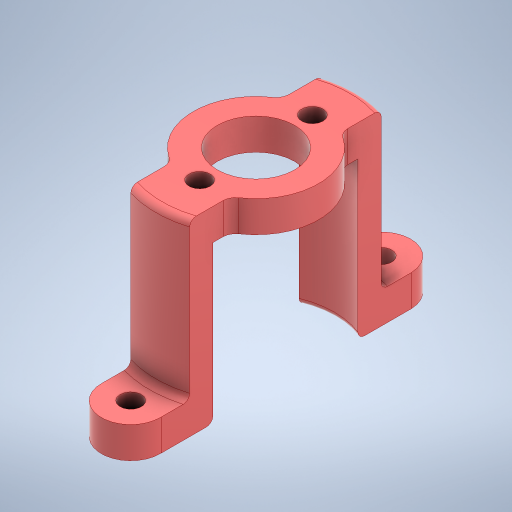
# Autodesk Inventor part: Th_3D_hn_1
Saved by Autodesk Inventor 2023 (Build 270158000, 158)
## iProperties
Created: 2020-11-15
Part Number: Th_3D_hn_1
Material: ABS プラスチック
Document SubType Name: Modeling
Designer: Haruka
Density: 1.06 g/cm^3
Appearance: 滑らか - 赤
Author: Haruka
Autodesk Inventor part; units mm, degrees
ref_plane "YZ Plane" through (0, 0, 0) normal (1, 0, 0) x (0, 1, 0)
ref_plane "XZ Plane" through (0, 0, 0) normal (0, 1, 0) x (-1, 0, 0)
ref_plane "XY Plane" through (0, 0, 0) normal (0, 0, 1) x (1, 0, 0)
sketch "スケッチ1" plane through (0, 0, 0) normal (0, 1, 0) x (-1, 0, 0)
  line L0 (0, 0) -> (0, -20) construction
  line L1 (0, 0) -> (0, 20) construction
  circle A0 centre (0, 20) radius 1.7
  circle A1 centre (0, -20) radius 1.7
  circle A2 centre (0, 20) radius 4.7
  circle A3 centre (0, -20) radius 4.7
  line L2 (4.698231, 19.871077) -> (4.7, -19.999792)
  line L3 (-4.697377, 19.843003) -> (-4.697377, -20.156997)
  circle A4 centre (0, 0) radius 12.5
  point P0 (-4.697377, 11.58381)
  point P1 (4.698599, 11.583314)
  point P2 (4.699627, -11.582897)
  point P3 (-4.697377, -11.58381)
  dimension "d0" = 20
  dimension "d1" = 20
  dimension "d2" = 3.4
  dimension "d3" = 3.4
  dimension "d5" = 3
  dimension "d6" = 3
  dimension "d7" = 25
  constraints: 8 end point, 5 centre point, 4 point on circle, 3 coincident, 3 vertical, 1 tangent
  measures "d0" distance of L0.start L0.end
  measures "d1" distance of L0.start L1.end
  measures "d2" diameter of A0
  measures "d3" diameter of A1
  measures "d5" radial gap between concentric circles of A0 A2
  measures "d6" radial gap between concentric circles of A3 A1
  measures "d7" diameter of A4
sketch "スケッチ1 outline for 押し出し1" plane through (0, 0, 0) normal (0, 1, 0) x (-1, 0, 0)
  arc A0 (-4.697377, 11.58381) -> (4.698599, 11.583314) centre (0, 0) cw
  line L0 (-4.697377, 19.843003) -> (-4.697377, 11.58381)
  line L1 (4.698599, 11.583314) -> (4.698231, 19.871077)
  arc A1 (4.698231, 19.871077) -> (-4.697377, 19.843003) centre (0, 20) ccw
  circle A2 centre (0, 20) radius 1.7
  arc A3 (-4.697377, -20.156997) -> (4.7, -19.999792) centre (0, -20) ccw
  line L2 (-4.697377, -11.58381) -> (-4.697377, -20.156997)
  line L3 (4.7, -19.999792) -> (4.699627, -11.582897)
  arc A4 (4.699627, -11.582897) -> (-4.697377, -11.58381) centre (0, 0) cw
  circle A5 centre (0, -20) radius 1.7
extrude "押し出し1" add sketch "スケッチ1 outline for 押し出し1" along normal blind 5
sketch "スケッチ2" plane through (0, 5, 0) normal (0, 1, 0) x (1, 0, 0)
  line L0 (-4.698599, -11.583314) -> (-4.698231, -19.871077)
  arc A0 (-4.698231, -19.871077) -> (4.697377, -19.843003) centre (0, -20) ccw
  line L1 (4.697377, -19.843003) -> (4.697377, -11.58381)
  arc A1 (-4.698599, -11.583314) -> (4.697377, -11.58381) centre (0, 0) ccw
  circle A2 centre (0, -20) radius 1.7
  arc A3 (4.697377, 20.156997) -> (-4.7, 19.999792) centre (0, 20) ccw
  line L2 (-4.7, 19.999792) -> (-4.699627, 11.582897)
  arc A4 (4.697377, 11.58381) -> (-4.699627, 11.582897) centre (0, 0) ccw
  line L3 (4.697377, 11.58381) -> (4.697377, 20.156997)
  circle A5 centre (0, 20) radius 1.7
  circle A6 centre (0, 0) radius 16
  point P0 (4.697377, 15.294922)
  point P1 (-4.699791, 15.294181)
  point P2 (-4.698434, -15.294598)
  point P3 (4.697377, -15.294922)
  dimension "d10" = 32
  constraints: 1 centre point, 1 coincident
  measures "d10" diameter of A6
extrude "押し出し2" add sketch "スケッチ2" along normal blind 20 contours A1 L1 A6 L0 | A6 L3 A4 L2
sketch "スケッチ3" plane through (0, 25, 0) normal (0, 1, 0) x (1, 0, 0)
  line L0 (-4.698599, -11.583314) -> (-4.698434, -15.294598)
  arc A0 (-4.698434, -15.294598) -> (4.697377, -15.294922) centre (0, 0) ccw
  line L1 (4.697377, -15.294922) -> (4.697377, -11.58381)
  arc A1 (-4.698599, -11.583314) -> (4.697377, -11.58381) centre (0, 0) ccw
  line L2 (-4.699791, 15.294181) -> (-4.699627, 11.582897)
  arc A2 (4.697377, 11.58381) -> (-4.699627, 11.582897) centre (0, 0) ccw
  line L3 (4.697377, 11.58381) -> (4.697377, 15.294922)
  arc A3 (4.697377, 15.294922) -> (-4.699791, 15.294181) centre (0, 0) ccw
  line L4 (-4.6, -11.583314) -> (-4.6, 11.582897)
  line L5 (4.697377, -11.58381) -> (4.697377, 11.58381)
  circle A4 centre (0, 0) radius 10
  point P0 (-4.699504, 8.826928)
  point P1 (-4.698721, -8.827345)
  point P2 (4.697377, -8.82806)
  point P3 (4.697377, 8.82806)
  dimension "d16" = 20
  constraints: 2 end point, 1 centre point, 1 coincident, 1 collinear, 3 other
  measures "d16" diameter of A4
sketch "スケッチ3 outline for 押し出し3" plane through (0, 25, 0) normal (0, 1, 0) x (1, 0, 0)
  arc A0 (4.697377, 15.294922) -> (-4.699791, 15.294181) centre (0, 0) ccw
  line L0 (-4.699791, 15.294181) -> (-4.699504, 8.826928)
  arc A1 (-4.699504, 8.826928) -> (-4.698721, -8.827345) centre (0, 0) ccw
  line L1 (-4.698721, -8.827345) -> (-4.698434, -15.294598)
  arc A2 (-4.698434, -15.294598) -> (4.697377, -15.294922) centre (0, 0) ccw
  line L2 (4.697377, -15.294922) -> (4.697377, -8.82806)
  arc A3 (4.697377, -8.82806) -> (4.697377, 8.82806) centre (0, 0) ccw
  line L3 (4.697377, 8.82806) -> (4.697377, 15.294922)
extrude "押し出し3" add sketch "スケッチ3 outline for 押し出し3" along normal blind 5
sketch "スケッチ5" plane through (0, 30, 0) normal (0, 1, 0) x (1, 0, 0)
  circle A0 centre (0, 0) radius 6
  line L0 (0, 0) -> (0, 9)
  line L1 (0, 9) -> (0, -9)
  dimension "d18" = 12
  dimension "d19" = 9
  dimension "d20" = 18
  constraints: 4 coincident, 4 end point, 1 centre point, 1 point on line, 1 vertical
  measures "d18" diameter of A0
  measures "d19" distance of L0.start L0.end
  measures "d20" distance of L0.end L1.end
hole "穴1" at (0, 30, -9) at (0, 30, 9) direction (0, -1, 0) diameter 3.4 end through all
sketch "スケッチ6" plane through (0, 30, 0) normal (0, 1, 0) x (1, 0, 0)
  point P0 (0, 0)
  point P1 (0, 0)
  constraints: 1 coincident
hole "穴2" at (0, 30, 0) direction (0, -1, 0) diameter 12.35 end through all
fillet "フィレット3" radius 2 4 edges at (-4.6987, 27.5, 8.8273) (-4.6995, 27.5, -8.8269) (4.6974, 27.5, 8.8281) (4.6974, 27.5, -8.8281)
fillet "フィレット4" radius 1 6 edges at (-0.0006, 30, 16) (-0.0013, 30, -16) (-0.0007, 0, 12.5) (-0.0012, 0, -12.5) (-0.0006, 5, 16) (-0.0013, 5, -16)
